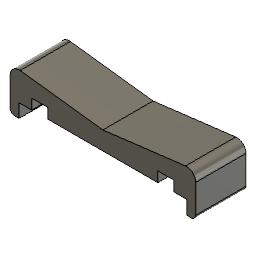
CalibrationAligner (Autodesk Fusion 360 design; units mm, degrees)
Autodesk Fusion 360 part; units mm, degrees
sketch "Sketch1" plane through (0, 0, 0) normal (0, 0, 1) x (1, 0, 0)
  line L0 (-40.65, 0) -> (40.65, 0)
  line L1 (40.65, 0) -> (40.65, 13)
  line L2 (40.65, 13) -> (0, 8)
  line L3 (0, 8) -> (-40.65, 13)
  line L4 (-40.65, 13) -> (-40.65, 0)
  line L5 (0, 8) -> (0, 0) construction
  dimension "d1" = 13
  dimension "d2" = 8
  dimension "d3" = 81.3
  constraint vertical L4
  constraint horizontal L0
  constraint vertical L1
  constraint midpoint L0 L5.end
  constraint vertical L5
  constraint equal L2 L3
  constraint equal L1 L4
  constraint coincident L5.end origin
  measures "d1" distance of L0.start L3.end
  measures "d2" distance of L2.end L5.end
  measures "d3" distance of L0.start L0.end
extrude "Extrude1" add sketch "Sketch1" along normal blind 22
sketch "Sketch2" plane through (0, 0, 0) normal (0, 0, -1) x (-1, 0, 0)
  line L0 (40.65, 0) -> (40.65, 13)
  line L1 (40.65, 13) -> (0, 8)
  line L2 (0, 8) -> (-40.65, 13)
  line L3 (-40.65, 13) -> (-40.65, 0)
  line L4 (-40.65, 0) -> (40.65, 0)
  line L5 (24.05, 4.5) -> (31.05, 4.5)
  line L6 (31.05, 4.5) -> (31.05, 0)
  line L7 (31.05, 0) -> (24.05, 0)
  line L8 (24.05, 0) -> (24.05, 4.5)
  line L9 (18.6, 10.2878) -> (18.6, 0) construction
  line L10 (36.5, 12.4895) -> (36.5, 0)
  line L11 (0, 8) -> (0, 0) construction
  line L12 (-24.05, 0) -> (-24.05, 4.5)
  line L13 (-24.05, 4.5) -> (-31.05, 4.5)
  line L14 (-31.05, 0) -> (-24.05, 0)
  line L15 (-31.05, 4.5) -> (-31.05, 0)
  point P0 (27.55, 0)
  dimension "d7" = 7
  dimension "d9" = 8.95
  dimension "d10" = 4.5
  dimension "d11" = 4.15
  dimension "d12" = 17.9
  constraint horizontal L5
  constraint vertical L6
  constraint horizontal L7
  constraint vertical L8
  constraint coincident L1 L9.start
  constraint coincident L4 L9.end
  constraint vertical L9
  constraint coincident L4 P0
  constraint midpoint L7 P0
  constraint coincident L1 L10.start
  constraint coincident L4 L10.end
  constraint perpendicular L4 L10
  constraint coincident L1.end L2.start
  constraint coincident L11.end origin
  constraint symmetric L5.start L11 L12.end
  constraint symmetric L5.end L11 L13.end
  constraint symmetric L6.end L11 L14.start
  constraint symmetric L7.end L11 L12.start
  measures "d7" distance of L6.end L7.end
  measures "d9" distance of L9.end P0
  measures "d10" distance of L5.end L6.end
  measures "d11" distance of L0 L10
  measures "d12" distance of L9 L10
extrude "Extrude2" cut sketch "Sketch2" against normal blind 22 contours L4 L5 L6 L7 L8 | L4 L12 L13 L14 L15
sketch "Sketch3" plane through (0, 0, 0) normal (0, 0, -1) x (-1, 0, 0)
  line L0 (31.05, 4.5) -> (31.05, 0)
  line L1 (31.05, 0) -> (40.65, 0)
  line L2 (40.65, 0) -> (40.65, 13)
  line L3 (40.65, 13) -> (0, 8)
  line L4 (0, 8) -> (-40.65, 13)
  line L5 (-40.65, 13) -> (-40.65, 0)
  line L6 (-40.65, 0) -> (-31.05, 0)
  line L7 (-31.05, 0) -> (-31.05, 4.5)
  line L8 (-31.05, 4.5) -> (-24.05, 4.5)
  line L9 (-24.05, 4.5) -> (-24.05, 0)
  line L10 (-24.05, 0) -> (24.05, 0)
  line L11 (24.05, 0) -> (24.05, 4.5)
  line L12 (24.05, 4.5) -> (31.05, 4.5)
  line L13 (0, 8) -> (0, 0) construction
  line L14 (40.65, 0) -> (36.65, 0)
  line L15 (36.65, 0) -> (36.65, -6)
  line L16 (36.65, -6) -> (40.65, -6)
  line L17 (40.65, -6) -> (40.65, 0)
  line L18 (-36.65, 0) -> (-36.65, -6)
  line L19 (-36.65, -6) -> (-40.65, -6)
  line L20 (-40.65, 0) -> (-36.65, 0)
  line L21 (-40.65, -6) -> (-40.65, 0)
  dimension "d15" = 4
  dimension "d16" = 6
  constraint coincident L3.end L4.start
  constraint coincident L13.end origin
  constraint horizontal L14
  constraint vertical L15
  constraint horizontal L16
  constraint vertical L17
  constraint coincident L1.end L2.start
  constraint symmetric L13 L1.end L5.end
  constraint symmetric L13 L14.end L18.start
  constraint symmetric L13 L15.end L18.end
  constraint symmetric L13 L16.end L19.end
  measures "d15" distance of L15.end L16.end
  measures "d16" distance of L1.end L16.end
extrude "Extrude3" add sketch "Sketch3" against normal blind 22 contours L1 L14 L15 L16 L17 | L6 L18 L19 L20 L21
fillet "Fillet1" radius 4 2 edges at (-40.65, 13, 11) (40.65, 13, 11)
fillet "Fillet2" radius 2 2 edges at (40.65, -6, 11) (-40.65, -6, 11)
equation "d3 = 73 mm + 2 * tolerance + ( 2 * 4 ) * 1 mm"
equation "tolerance = 0.15 mm"
equation "d9 = ( 17.9 / 2 ) * 1 mm"
equation "d11 = 4 mm + tolerance"
